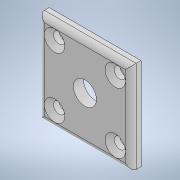
# Autodesk Inventor part: Крышка поворотного кулака
Saved by Autodesk Inventor 2020 (Build 240168000, 168)
## iProperties
Created: 2021-04-25
Part Number: Крышка поворотного кулака
Material: Типовые
Document SubType Name: Modeling
Designer: Антон
Density: 1 g/cm^3
Appearance: По умолчанию
Author: Антон
Autodesk Inventor part; units mm, degrees
ref_plane "YZ Plane" through (0, 0, 0) normal (1, 0, 0) x (0, 1, 0)
ref_plane "XZ Plane" through (0, 0, 0) normal (0, 1, 0) x (-1, 0, 0)
ref_plane "XY Plane" through (0, 0, 0) normal (0, 0, 1) x (1, 0, 0)
sketch "Эскиз1" plane through (0, 0, 0) normal (0, 0, 1) x (1, 0, 0)
  line L0 (0, 0) -> (18, 0)
  line L1 (18, 0) -> (18, 18)
  line L2 (18, 18) -> (0, 18)
  line L3 (0, 18) -> (0, 0)
  dimension "d0" = 18
  dimension "d1" = 18
  constraints: 8 end point, 2 parallel, 1 horizontal, 1 perpendicular
  measures "d0" distance of L2.end L1.end
  measures "d1" distance of L1.end L0.end
extrude "Выдавливание1" add sketch "Эскиз1" along normal blind 2
sketch "Эскиз8" plane through (0, 0, 2) normal (0, 0, 1) x (1, 0, 0)
  line L0 (18, 18) -> (0, 18) construction
  line L1 (0, 0) -> (18, 18) construction
  line L2 (0, 0) -> (18, 0) construction
  line L3 (0, 18) -> (18, 0) construction
  circle A0 centre (9, 9) radius 2.25
  dimension "d38" = 4.5
  constraints: 4 end point, 1 centre point, 1 midpoint
  measures "d38" diameter of A0
extrude "Выдавливание5" cut sketch "Эскиз8" against normal through all
sketch "Эскиз9" plane through (0, 0, 2) normal (0, 0, 1) x (1, 0, 0)
  circle A0 centre (9, 9) radius 2.25 construction
  circle A1 centre (9, 9) radius 4.1 construction
  line L0 (0, 18) -> (0, 0) construction
  line L1 (0, 18) -> (6.1009, 11.8991) construction
  line L2 (18, 0) -> (18, 18) construction
  line L3 (18, 18) -> (11.8991, 11.8991) construction
  line L4 (0, 0) -> (6.1009, 6.1009) construction
  line L5 (0, 0) -> (18, 0) construction
  line L6 (18, 0) -> (11.8991, 6.1009) construction
  point P0 (3.0504, 14.9496)
  point P1 (14.9496, 14.9496)
  point P2 (3.0504, 3.0504)
  point P3 (14.9496, 3.0504)
  dimension "d41" = 8.2
  constraints: 8 end point, 4 midpoint, 4 point on circle, 2 collinear, 1 centre point, 1 coincident
  measures "d41" diameter of A1
hole "Отверстие4" at (3.0504, 14.9496, 2) at (3.0504, 3.0504, 2) at (14.9496, 3.0504, 2) at (14.9496, 14.9496, 2) direction (0, 0, -1) diameter 2.2 end through all countersink diameter 4 countersink angle 90
fillet "Сопряжение2" radius 1.05 4 edges at (9, 0, 2) (0, 9, 2) (9, 18, 2) (18, 9, 2)
